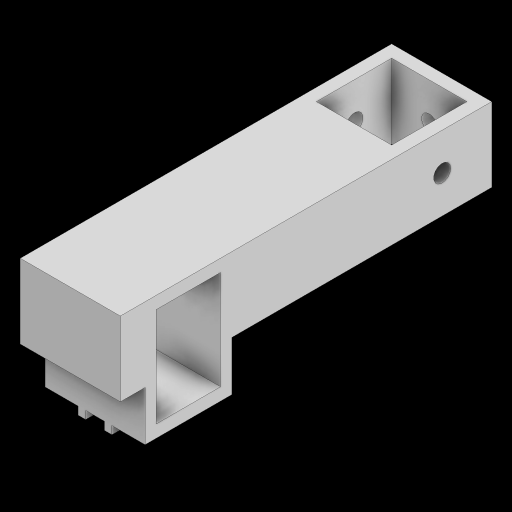
# Autodesk Inventor part: lever_support
Saved by Autodesk Inventor 2023 (Build 270158000, 158)
## iProperties
Created: 2024-07-03
Part Number: lever_support
Material: 일반
Document SubType Name: Modeling
Designer: OMS55
Density: 1 g/cm^3
Appearance: 기본값
Author: OMS55
Autodesk Inventor part; units mm, degrees
ref_plane "YZ Plane" through (0, 0, 0) normal (1, 0, 0) x (0, 1, 0)
ref_plane "XZ Plane" through (0, 0, 0) normal (0, 1, 0) x (-1, 0, 0)
ref_plane "XY Plane" through (0, 0, 0) normal (0, 0, 1) x (1, 0, 0)
sketch "스케치1" plane through (0, 0, 0) normal (0, 1, 0) x (-1, 0, 0)
  line L0 (40.4, 0) -> (0, 0)
  line L1 (0, 0) -> (0, -150)
  line L2 (0, -150) -> (40.4, -150)
  line L3 (40.4, -150) -> (40.4, 0)
  line L4 (35.4, -114.6) -> (5, -114.6)
  line L5 (5, -114.6) -> (5, -145)
  line L6 (5, -145) -> (35.4, -145)
  line L7 (35.4, -145) -> (35.4, -114.6)
  line L8 (20.2, -114.6) -> (20.2, -145) construction
  line L9 (35.4, -129.8) -> (5, -129.8) construction
  line L10 (35.65, -10) -> (4.75, -10)
  line L11 (4.75, -10) -> (4.75, -80)
  line L12 (4.75, -80) -> (35.65, -80)
  line L13 (35.65, -80) -> (35.65, -10)
  point P0 (20.2, -150)
  dimension "d0" = 30.4
  dimension "d1" = 30.4
  dimension "d2" = 5
  dimension "d3" = 5
  dimension "d4" = 5
  dimension "d5" = 70
  dimension "d6" = 4.75
  dimension "d7" = 4.75
  dimension "d8" = 10
  dimension "d9" = 150
  constraints: 28 end point, 6 parallel, 5 midpoint, 3 horizontal, 3 perpendicular, 1 coincident
  measures "d0" distance of L6.end L4.start
  measures "d1" distance of L5.end L6.end
  measures "d2" distance between parallel lines of L7 L3
  measures "d3" distance between parallel lines of L6 L2
  measures "d4" distance between parallel lines of L1 L5
  measures "d5" distance of L12.end L10.start
  measures "d6" distance between parallel lines of L3 L13
  measures "d7" distance between parallel lines of L1 L11
  measures "d8" distance between parallel lines of L0 L10
  measures "d9" distance from line of point (20.2, -150) L0
extrude "돌출1" add sketch "스케치1" along normal blind 30
sketch "스케치2" plane through (0, 0, 0) normal (1, 0, 0) x (0, 0, -1)
  circle A0 centre (130, 15) radius 3.45
  line L0 (150, 0) -> (150, 30) projected
  line L1 (0, 30) -> (150, 30) projected
  point P0 (0, 0)
  dimension "d12" = 20
  dimension "d13" = 15
  dimension "d14" = 6.9
  constraints: 1 centre point
  measures "d12" distance from line of L0 A0.centre
  measures "d13" distance from line of L1 A0.centre
  measures "d14" diameter of A0
extrude "돌출2" cut sketch "스케치2" against normal blind 50
sketch "스케치3" plane through (0, 0, -150) normal (0, 0, -1) x (-1, 0, 0)
  circle A0 centre (20.2, 15) radius 3.15
  line L0 (0, 30) -> (40.4, 30) projected
  line L1 (40.4, 0) -> (40.4, 30) projected
  point P0 (0, 0)
  point P1 (20.2, 30)
  point P2 (40.4, 15)
  dimension "d17" = 6.3
  constraints: 2 midpoint, 1 centre point, 1 horizontal alignment, 1 vertical alignment
  measures "d17" diameter of A0
extrude "돌출3" cut sketch "스케치3" against normal blind 10
extrude "돌출5" add sketch "스케치1" along normal up to surface (30 mm away) contours L13 L12 L11 L10
sketch "스케치5" plane through (0, 0, 0) normal (0, -1, 0) x (1, 0, 0)
  line L0 (-4.75, -10) -> (-35.65, -10)
  line L1 (-35.65, -10) -> (-35.65, -45)
  line L2 (-35.65, -45) -> (-4.75, -45)
  line L3 (-4.75, -45) -> (-4.75, -10)
  line L4 (-4.75, -10) -> (-4.75, -80) projected
  line L5 (-35.65, -10) -> (-4.75, -10) projected
  line L6 (0, -10) -> (-40.4, -10)
  line L7 (-40.4, -10) -> (-40.4, -45)
  line L8 (-40.4, -45) -> (0, -45)
  line L9 (0, -45) -> (0, -10)
  line L10 (0, 0) -> (0, -150) projected
  line L11 (-40.4, -150) -> (-40.4, 0) projected
  line L12 (-40.4, -150) -> (-40.4, 0) projected
  point P0 (-4.75, -45)
  dimension "d27" = 35
  constraints: 16 end point, 3 collinear, 2 parallel, 2 point on line, 1 horizontal, 1 perpendicular
  measures "d27" distance of L2.end L0.start
extrude "돌출6" add sketch "스케치5" along normal blind 20
sketch "스케치6" plane through (0, 0, -150) normal (1, 0, 0) x (0, 0, -1)
  line L0 (-135.5, -15) -> (-109.5, -15)
  line L1 (-109.5, -15) -> (-109.5, 25)
  line L2 (-109.5, 25) -> (-135.5, 25)
  line L3 (-135.5, 25) -> (-135.5, -15)
  line L4 (-150, 30) -> (0, 30) projected
  line L5 (-105, -20) -> (-140, -20) projected
  line L6 (-140, 0) -> (-140, -20) projected
  point P0 (-150, 0)
  dimension "d30" = 5
  dimension "d31" = 5
  dimension "d32" = 26
  dimension "d33" = 4.5
  constraints: 8 end point, 2 parallel, 1 horizontal, 1 perpendicular
  measures "d30" distance between parallel lines of L4 L2
  measures "d31" distance between parallel lines of L5 L0
  measures "d32" distance between parallel lines of L1 L3
  measures "d33" distance between parallel lines of L3 L6
extrude "돌출7" cut sketch "스케치6" against normal up to surface (40.4 mm away)
sketch "스케치7" plane through (0, -15, -14.5) normal (0, 1, 0) x (1, 0, 0)
  circle A0 centre (-20.2, 14.3) radius 1.45
  line L0 (0, -4.5) -> (-40.4, -4.5) projected
  line L1 (-40.4, 30.5) -> (0, 30.5) projected
  point P0 (0, -14.5)
  point P1 (-20.2, 30.5)
  dimension "d36" = 2.9
  dimension "d37" = 18.8
  constraints: 1 centre point, 1 midpoint, 1 vertical alignment
  measures "d36" diameter of A0
  measures "d37" distance from line of A0.centre L0
extrude "돌출8" cut sketch "스케치7" against normal blind 10
sketch "스케치8" plane through (0, -20, 0) normal (0, -1, 0) x (1, 0, 0)
  line L0 (0, -10) -> (-40.4, -10) projected
  line L1 (-13.4, -10) -> (-16.4, -10)
  line L2 (-16.4, -10) -> (-16.4, -45)
  line L3 (-16.4, -45) -> (-13.4, -45)
  line L4 (-13.4, -45) -> (-13.4, -10)
  line L5 (-24, -10) -> (-27, -10)
  line L6 (-27, -10) -> (-27, -45)
  line L7 (-27, -45) -> (-24, -45)
  line L8 (-24, -45) -> (-24, -10)
  line L9 (-40.4, -45) -> (0, -45) projected
  circle A0 centre (-20.2, -28.8) radius 1.45 projected
  point P0 (0, 0)
  dimension "d40" = 7.6
  dimension "d41" = 3.8
  dimension "d42" = 3
  dimension "d43" = 3
  constraints: 16 end point, 4 parallel, 2 collinear, 2 horizontal, 2 perpendicular, 2 point on line
  measures "d40" distance between parallel lines of L8 L2
  measures "d41" distance from line of L8 A0.centre
  measures "d42" distance between parallel lines of L2 L4
  measures "d43" distance between parallel lines of L6 L8
extrude "돌출9" add sketch "스케치8" along normal blind 3.2 contours L4 L3 L2 L0 | L8 L7 L6 L0
